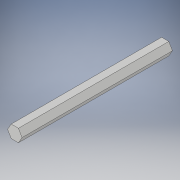
# Autodesk Inventor part: Drivetrain_hex_shaft
Saved by Autodesk Inventor 2018 (Build 220112000, 112)
## iProperties
Created: 2018-09-05
Part Number: Drivetrain_hex_shaft
Material: Generic
Document SubType Name: Modeling
Designer: baoan
Density: 1 g/cm^3
Appearance: Default
Author: baoan
Autodesk Inventor part; units mm, degrees
ref_plane "YZ Plane" through (0, 0, 0) normal (1, 0, 0) x (0, 1, 0)
ref_plane "XZ Plane" through (0, 0, 0) normal (0, 1, 0) x (-1, 0, 0)
ref_plane "XY Plane" through (0, 0, 0) normal (0, 0, 1) x (1, 0, 0)
sketch "Sketch1" plane through (0, 0, 0) normal (0, 0, 1) x (1, 0, 0)
  line L0 (-3.6703, 6.3571) -> (3.6703, 6.3571)
  line L1 (3.6703, 6.3571) -> (7.3406, 0)
  line L2 (7.3406, 0) -> (3.6703, -6.3571)
  line L3 (3.6703, -6.3571) -> (-3.6703, -6.3571)
  line L4 (-3.6703, -6.3571) -> (-7.3406, 0)
  line L5 (-7.3406, 0) -> (-3.6703, 6.3571)
  point P0 (0, 0)
  point P1 (0, 0)
  dimension "d0" = 7.3406
  constraints: 12 end point, 1 coincident, 1 horizontal, 13 other
  measures "d0" distance of L0.start L0.end
extrude "Extrusion1" add sketch "Sketch1" along normal mid plane 152.4
body "Solid1"
